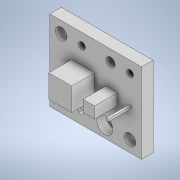
# Autodesk Inventor part: Тестовая модель (Валы, столбы, подшипники)
Saved by Autodesk Inventor 2020 (Build 240168000, 168)
## iProperties
Created: 2021-03-07
Part Number: Тестовая модель (Валы, столбы, подшипники)
Material: Типовые
Document SubType Name: Modeling
Designer: Антон
Density: 1 g/cm^3
Appearance: По умолчанию
Author: Антон
Autodesk Inventor part; units mm, degrees
ref_plane "YZ Plane" through (0, 0, 0) normal (1, 0, 0) x (0, 1, 0)
ref_plane "XZ Plane" through (0, 0, 0) normal (0, 1, 0) x (-1, 0, 0)
ref_plane "XY Plane" through (0, 0, 0) normal (0, 0, 1) x (1, 0, 0)
sketch "Эскиз1" plane through (0, 0, 0) normal (0, 0, 1) x (1, 0, 0)
  line L0 (0, 0) -> (40, 0)
  line L1 (40, 0) -> (40, 35)
  line L2 (40, 35) -> (0, 35)
  line L3 (0, 35) -> (0, 0)
  line L4 (0, 17.5) -> (40, 17.5)
  line L5 (5, 5) -> (35, 5)
  line L6 (35, 5) -> (35, 30)
  line L7 (35, 30) -> (5, 30)
  line L8 (5, 30) -> (5, 5)
  line L9 (5, 5) -> (35, 30) construction
  line L10 (35, 5) -> (5, 30) construction
  circle A0 centre (5, 30) radius 2.5
  line L11 (5, 30) -> (14, 30)
  circle A1 centre (14, 30) radius 1.5
  line L12 (2.5, 2.5) -> (7.5, 2.5)
  line L13 (7.5, 2.5) -> (7.5, 7.5)
  line L14 (7.5, 7.5) -> (2.5, 7.5)
  line L15 (2.5, 7.5) -> (2.5, 2.5)
  line L16 (2.5, 2.5) -> (7.5, 7.5) construction
  line L17 (7.5, 2.5) -> (2.5, 7.5) construction
  line L18 (5, 5) -> (13.5, 5)
  line L19 (12.5, 6) -> (14.5, 6)
  line L20 (14.5, 6) -> (14.5, 4)
  line L21 (14.5, 4) -> (12.5, 4)
  line L22 (12.5, 4) -> (12.5, 6)
  line L23 (12.5, 6) -> (14.5, 4) construction
  line L24 (14.5, 6) -> (12.5, 4) construction
  point P0 (20, 17.5)
  dimension "d0" = 40
  dimension "d1" = 35
  dimension "d2" = 30
  dimension "d3" = 25
  dimension "d4" = 5
  dimension "d5" = 9
  dimension "d6" = 3
  dimension "d7" = 5
  dimension "d8" = 5
  dimension "d9" = 8.5
  dimension "d10" = 2
  dimension "d11" = 2
  constraints: 50 end point, 9 midpoint, 8 parallel, 4 horizontal, 4 perpendicular, 2 centre point, 2 coincident, 2 point on line
  measures "d0" distance of L2.end L1.end
  measures "d1" distance of L1.end L0.end
  measures "d2" distance of L7.end L6.end
  measures "d3" distance of L6.end L5.end
  measures "d4" diameter of A0
  measures "d5" distance of L11.start L11.end
  measures "d6" diameter of A1
  measures "d7" distance of L14.end L13.end
  measures "d8" distance of L13.end L12.end
  measures "d9" distance of L5.start L18.end
  measures "d10" distance of L20.end L21.end
  measures "d11" distance of L19.end L20.end
extrude "Выдавливание1" add sketch "Эскиз1" along normal blind 5 contours L3 L4 L8 L14 L15 L12 L13 L5 L22 L21 L20 L6 L1 L0 | L3 L2 L1 L4 L6 L7 A1 A0 L8 | L8 A0 L7 A1 L6 L4 | L4 L6 L5 L20 L19 L22 L13 L14 L8
sketch "Эскиз3" plane through (0, 0, 5) normal (0, 0, 1) x (1, 0, 0)
  line L0 (0, 35) -> (0, 0) projected
  line L1 (0, 17.5) -> (40, 17.5)
  line L2 (40, 0) -> (40, 35) projected
  line L3 (40, 0) -> (40, 35) projected
  line L4 (40, 35) -> (0, 35) projected
  line L5 (0, 35) -> (0, 0) projected
  line L6 (0, 0) -> (40, 0) projected
  line L7 (7.5, 7.5) -> (7.5, 2.5) projected
  line L8 (7.5, 2.5) -> (2.5, 2.5) projected
  line L9 (2.5, 2.5) -> (2.5, 7.5) projected
  line L10 (2.5, 7.5) -> (7.5, 7.5) projected
  line L11 (14.5, 4) -> (12.5, 4) projected
  line L12 (12.5, 4) -> (12.5, 6) projected
  line L13 (12.5, 6) -> (14.5, 6) projected
  line L14 (14.5, 6) -> (14.5, 4) projected
  circle A0 centre (14, 30) radius 1.5 projected
  circle A1 centre (5, 30) radius 2.5 projected
  line L15 (5, 5) -> (35, 5)
  line L16 (35, 5) -> (35, 30)
  line L17 (35, 30) -> (5, 30)
  line L18 (5, 30) -> (5, 5)
  line L19 (5, 5) -> (35, 30) construction
  line L20 (35, 5) -> (5, 30) construction
  line L21 (34.5, 17) -> (35.5, 17)
  line L22 (35.5, 17) -> (35.5, 18)
  line L23 (35.5, 18) -> (34.5, 18)
  line L24 (34.5, 18) -> (34.5, 17)
  line L25 (34.5, 17) -> (35.5, 18) construction
  line L26 (35.5, 17) -> (34.5, 18) construction
  line L27 (35, 17.5) -> (27, 17.5)
  line L28 (24.5, 15) -> (29.5, 15)
  line L29 (29.5, 15) -> (29.5, 20)
  line L30 (29.5, 20) -> (24.5, 20)
  line L31 (24.5, 20) -> (24.5, 15)
  line L32 (24.5, 15) -> (29.5, 20) construction
  line L33 (29.5, 15) -> (24.5, 20) construction
  line L34 (27, 17.5) -> (14.5, 17.5)
  line L35 (9.5, 12.5) -> (19.5, 12.5)
  line L36 (19.5, 12.5) -> (19.5, 22.5)
  line L37 (19.5, 22.5) -> (9.5, 22.5)
  line L38 (9.5, 22.5) -> (9.5, 12.5)
  line L39 (9.5, 12.5) -> (19.5, 22.5) construction
  line L40 (19.5, 12.5) -> (9.5, 22.5) construction
  line L41 (24.5, 20) -> (29.5, 20)
  line L42 (29.5, 20) -> (29.5, 15)
  line L43 (29.5, 15) -> (24.5, 15)
  line L44 (24.5, 15) -> (24.5, 20)
  point P0 (20, 17.5)
  dimension "d14" = 35
  dimension "d15" = 40
  dimension "d16" = 30
  dimension "d17" = 25
  dimension "d18" = 1
  dimension "d19" = 1
  dimension "d20" = 8
  dimension "d21" = 5
  dimension "d22" = 5
  dimension "d23" = 12.5
  dimension "d24" = 10
  dimension "d25" = 10
  constraints: 62 end point, 12 midpoint, 10 parallel, 5 horizontal, 5 perpendicular, 2 point on line
  measures "d14" distance of L2.start L2.end
  measures "d15" distance of L3.end L4.end
  measures "d16" distance of L17.end L16.end
  measures "d17" distance of L16.end L15.end
  measures "d18" distance of L23.end L22.end
  measures "d19" distance of L22.end L21.end
  measures "d20" distance of L27.start L27.end
  measures "d21" distance of L30.end L29.end
  measures "d22" distance of L29.end L28.end
  measures "d23" distance of L27.end L34.end
  measures "d24" distance of L37.end L36.end
  measures "d25" distance of L36.end L35.end
extrude "Выдавливание2" add sketch "Эскиз3" along normal blind 10 contours L38 L37 L36 L1 | L1 L36 L35 L38 | L22 L21 L16 L1 | L1 L16 L23 L22 | L16 L21 L24 L1 | L1 L24 L23 L16 | L31 L30 L29 L1 | L1 L29 L28 L31
sketch "Эскиз4" plane through (0, 0, 5) normal (0, 0, 1) x (1, 0, 0)
  line L0 (34.5, 17) -> (34.5, 18) projected
  line L1 (34.5, 18) -> (35.5, 18) projected
  line L2 (35.5, 18) -> (35.5, 17) projected
  line L3 (35.5, 17) -> (34.5, 17) projected
  line L4 (19.5, 22.5) -> (19.5, 12.5) projected
  line L5 (19.5, 12.5) -> (9.5, 12.5) projected
  line L6 (9.5, 12.5) -> (9.5, 22.5) projected
  line L7 (9.5, 22.5) -> (19.5, 22.5) projected
  line L8 (24.5, 15) -> (24.5, 20) projected
  line L9 (24.5, 20) -> (29.5, 20) projected
  line L10 (29.5, 20) -> (29.5, 15) projected
  line L11 (29.5, 15) -> (24.5, 15) projected
  line L12 (0, 35) -> (0, 0) projected
  line L13 (0, 0) -> (40, 0) projected
  line L14 (40, 0) -> (40, 35) projected
  line L15 (40, 35) -> (0, 35) projected
  line L16 (2.5, 2.5) -> (2.5, 7.5) projected
  line L17 (2.5, 7.5) -> (7.5, 7.5) projected
  line L18 (7.5, 7.5) -> (7.5, 2.5) projected
  line L19 (7.5, 2.5) -> (2.5, 2.5) projected
  line L20 (12.5, 6) -> (14.5, 6) projected
  line L21 (14.5, 6) -> (14.5, 4) projected
  line L22 (14.5, 4) -> (12.5, 4) projected
  line L23 (12.5, 4) -> (12.5, 6) projected
  circle A0 centre (14, 30) radius 1.5 projected
  circle A1 centre (5, 30) radius 2.5 projected
  line L24 (0, 35) -> (0, 0) projected
  line L25 (0, 17.5) -> (40, 17.5)
  line L26 (40, 0) -> (40, 35) projected
  line L27 (5, 5) -> (35, 5)
  line L28 (35, 5) -> (35, 30)
  line L29 (35, 30) -> (5, 30)
  line L30 (5, 30) -> (5, 5)
  line L31 (5, 5) -> (35, 30) construction
  line L32 (35, 5) -> (5, 30) construction
  circle A2 centre (35, 30) radius 1.5
  line L33 (35, 30) -> (26.5, 30)
  circle A3 centre (26.5, 30) radius 2
  circle A4 centre (35, 5) radius 2.5
  line L34 (35, 5) -> (24, 5)
  circle A5 centre (24, 5) radius 3.5
  point P0 (20, 17.5)
  dimension "d28" = 30
  dimension "d29" = 25
  dimension "d30" = 35
  dimension "d31" = 40
  dimension "d32" = 3
  dimension "d33" = 8.5
  dimension "d34" = 4
  dimension "d35" = 5
  dimension "d36" = 11
  dimension "d37" = 7
  constraints: 18 end point, 5 midpoint, 4 centre point, 4 coincident, 2 parallel, 2 point on line, 1 horizontal, 1 perpendicular
  measures "d28" distance of L29.end L28.end
  measures "d29" distance of L28.end L27.end
  measures "d30" distance of L13.end L14.end
  measures "d31" distance of L14.end L12.start
  measures "d32" diameter of A2
  measures "d33" distance of L33.start L33.end
  measures "d34" diameter of A3
  measures "d35" diameter of A4
  measures "d36" distance of L34.start L34.end
  measures "d37" diameter of A5
extrude "Выдавливание3" cut sketch "Эскиз4" against normal blind 4 contours A4 L27 L28 | L28 L27 A4 | A2 L29 L28 | L28 L29 A2 | A5 L27 | L27 A5 | A3 L29 | L29 A3
sketch "Эскиз5" plane through (26.5, 30, 1) normal (0, 0, 1) x (1, 0, 0)
  circle A0 centre (0, 0) radius 2 projected
  circle A1 centre (8.5, 0) radius 1.5 projected
  circle A2 centre (-2.5, -25) radius 3.5 projected
  circle A3 centre (8.5, -25) radius 2.5 projected
  point P0 (-26.5, -30)
hole "Отверстие1" at (26.5, 30, 1) at (35, 30, 1) at (24, 5, 1) at (35, 5, 1) direction (0, 0, -1) diameter 2 end through all
